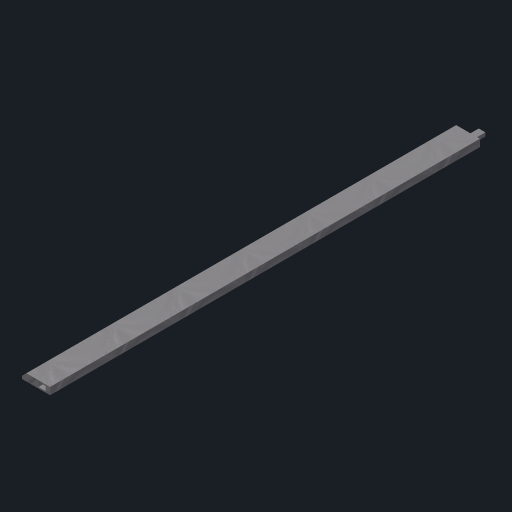
# Autodesk Inventor part: SEPARADOR
Saved by Autodesk Inventor 2024.3 (Build 283343000, 343)
## iProperties
Created: 2024-07-03
Part Number: SEPARADOR
Material: Steel, Mild, Welded
Document SubType Name: Modeling
Designer: Niler
Density: 7.85 g/cm^3
Appearance: Weld - Steel Mild
Author: Niler
Autodesk Inventor part; units mm, degrees
ref_plane "YZ Plane" through (0, 0, 0) normal (1, 0, 0) x (0, 1, 0)
ref_plane "XZ Plane" through (0, 0, 0) normal (0, 1, 0) x (-1, 0, 0)
ref_plane "XY Plane" through (0, 0, 0) normal (0, 0, 1) x (1, 0, 0)
sketch "Sketch1" plane through (0, 0, 0) normal (0, 1, 0) x (-1, 0, 0)
  line L0 (-9.75, 149.5) -> (9.75, 149.5)
  line L1 (9.75, 149.5) -> (9.75, -149.5)
  line L2 (9.75, -149.5) -> (-9.75, -149.5)
  line L3 (-9.75, -149.5) -> (-9.75, 149.5)
  line L4 (-9.75, 149.5) -> (9.75, -149.5) construction
  line L5 (9.75, 149.5) -> (-9.75, -149.5) construction
  point P0 (0, 0)
  dimension "d0" = 19.5
  dimension "d1" = 299
  constraints: 12 end point, 2 midpoint, 2 parallel, 1 horizontal, 1 perpendicular
  measures "d0" distance of L1.end L2.end
  measures "d1" distance of L0.end L1.end
extrude "Extrusion1" add sketch "Sketch1" along normal blind 5
chamfer "Chamfer1" distance 3 angle 45 1 edges at (-9.75, 5, 0)
sketch "Sketch2" plane through (-9.75, 0, 149.5) normal (0, 0, 1) x (1, 0, 0)
  line L0 (0, 2) -> (3, 5) projected
  line L1 (0, 0) -> (0, 2) projected
  line L2 (0, 0) -> (19.5, 0) projected
  line L3 (19.5, 0) -> (19.5, 5) projected
  line L4 (3, 5) -> (19.5, 5) projected
  line L5 (16.5, 4) -> (11.5, 4)
  line L6 (11.5, 4) -> (11.5, 1)
  line L7 (11.5, 1) -> (16.5, 1)
  line L8 (16.5, 1) -> (16.5, 4)
  line L9 (16.5, 4) -> (11.5, 1) construction
  line L10 (11.5, 4) -> (16.5, 1) construction
  point P0 (9.75, 0)
  point P1 (14, 2.5)
  point P2 (19.5, 2.5)
  dimension "d7" = 5
  dimension "d8" = 3
  dimension "d9" = 3
  constraints: 12 end point, 3 midpoint, 2 parallel, 1 horizontal, 1 horizontal alignment, 1 perpendicular
  measures "d7" distance of L7.end L6.end
  measures "d8" distance of L6.end L5.end
  measures "d9" distance between parallel lines of L8 L3
extrude "Extrusion2" cut sketch "Sketch2" against normal blind 7.1 contours L8 L7 L6 L5
sketch "Sketch3" plane through (9.75, 0, -149.5) normal (0, 0, -1) x (-1, 0, 0)
  line L0 (8, 1) -> (8, 4) projected
  line L1 (3, 1) -> (8, 1) projected
  line L2 (3, 4) -> (3, 1) projected
  line L3 (8, 4) -> (3, 4) projected
  line L4 (7.8, 1.2) -> (7.8, 3.8)
  line L5 (7.8, 3.8) -> (3.2, 3.8)
  line L6 (3.2, 3.8) -> (3.2, 1.2)
  line L7 (3.2, 1.2) -> (7.8, 1.2)
  point P0 (9.75, 0)
  dimension "d12" = 0.2
  constraints: 8 end point, 3 other
  measures "d12" distance between parallel lines of L1 L7
extrude "Extrusion3" add sketch "Sketch3" along normal blind 7 contours L7 L6 L5 L4
body "Solid1"
